Autodesk Fusion 360 part; units mm, degrees
(part 2 of 2)
  constraint perpendicular L106 L211
  constraint horizontal L241
  constraint coincident L210 L241.end
  constraint perpendicular L210 L242
  constraint coincident L210 L243.start
  constraint perpendicular L233 L243
  constraint coincident L233 L243.end
  constraint concentric A1 A243
  constraint concentric A4 A245
  constraint concentric A3 A246
  constraint tangent A134 L244
  constraint tangent L244 A247
  constraint tangent L245 A247
  constraint tangent L113 A248
  constraint tangent L116 A248
  constraint tangent L117 A249
  constraint tangent L120 A249
  constraint tangent L133 A250
  constraint tangent L132 A250
  constraint tangent L178 A251
  constraint tangent L177 A251
  constraint tangent L172 A252
  constraint tangent L171 A252
  constraint tangent L246 A253
  constraint tangent L185 A253
  constraint tangent L247 A254
  constraint tangent L248 A254
  constraint tangent L110 A255
  constraint tangent L242 A255
  constraint tangent L109 A256
  constraint tangent L110 A256
  constraint tangent L108 A257
  constraint tangent L241 A257
  constraint tangent L106 A258
  constraint tangent L107 A258
  measures "d1" diameter of A0
  measures "d2" diameter of A1
  measures "d3" diameter of A2
  measures "d4" diameter of A3
  measures "d5" diameter of A4
  measures "d9" diameter of A111
  measures "d12" diameter of A112
  measures "d255" diameter of A243
  measures "d256" diameter of A244
  measures "d257" diameter of A245
  measures "d259" diameter of A246
extrude "Extrude1" add sketch "mriya" along normal blind 10.6 contours L196 A199 L197 A200 L198 A201 L199 A202 L200 A203 L201 A204 L202 A205 L203 A206 L204 A207 L205 A208 L206 A209 L207 A210 L208 A211 L209 A212 L210 L211 A214 L212 A215 L213 A216 L214 A217 L215 A218 L216 A219 L217 A220 L218 L219 L220 A221 L221 A222 L222 L223 L224 L225 L226 L227 L228 L229 L230 L231 L232 L233 A224 L234 L235 L236 L237 L238 L239 A225 A226 A227 A228 A229 A230 A231 A232 L240 A233 A234 A235 A236 A237 A238 A239 A240 A241 A242 L243 picked at (-141.416666, 51.759867) makes body 1
extrude "Extrude2" add sketch "mriya" along normal blind 17.1 contours L210 A213 L211 L232 A223 L233 L240 L243 picked at (-5.283334, 44.5932) bodies 1
extrude "Extrude3" add sketch "mriya" along normal blind 3.7 contours L106 L107 L108 A113 L109 L110 L196 A199 L197 A200 L198 A201 L199 A202 L200 A203 L201 A204 L202 A205 L203 A206 L204 A207 L205 A208 L206 A209 L207 A210 L208 A211 L209 A212 L210 L211 A214 L212 A215 L213 A216 L214 A217 L215 A218 L216 A219 L217 A220 L241 L242 A255 A256 A257 A258 | L106 L107 L108 A113 L210 A213 L211 L241 A257 A258 | L109 L110 L210 L242 A255 A256 | A115 | A116 | A117 | A118 picked at (-84.826309, 24.168075) picked at (-7.216667, 50.959867) picked at (-7.216666, 8.059867) picked at (-64.728451, 82.79316) picked at (-45.728484, 78.29313) picked at (-25.071567, 2.493271) picked at (-44.071558, 4.793248) bodies 1
extrude "Extrude6" add sketch "mriya" along normal blind 1 from surface at 14.3 contours L106 L107 L108 A113 L210 A213 L211 L241 A257 A258 picked at (-7.216667, 50.959867) bodies 1
extrude "Extrude7" add sketch "mriya" along normal blind 1 from surface at 7.8 contours L109 L110 L210 L242 A255 A256 picked at (-7.216666, 8.059867) bodies 1
sketch "power-switch" plane through (-4.449999, 0, 0) normal (1, 0, 0) x (0, 1, 0)
  line L0 (19.1932, 0) -> (76.4932, 0)
  line L1 (76.4932, 0) -> (76.4932, 16.8)
  line L2 (76.4932, 16.8) -> (19.1932, 16.8)
  line L3 (19.1932, 16.8) -> (19.1932, 10.5)
  line L4 (36.0932, 5.1) -> (25.6932, 5.1)
  line L5 (25.6932, 5.1) -> (25.6932, 8)
  line L6 (25.6932, 8) -> (36.0932, 8)
  line L7 (36.0932, 8) -> (36.0932, 5.1)
  line L8 (37.4932, 3.55) -> (24.2932, 3.55)
  line L9 (23.8932, 3.95) -> (23.8932, 9.15)
  line L10 (24.2932, 9.55) -> (37.4932, 9.55)
  line L11 (37.8932, 9.15) -> (37.8932, 3.95)
  line L12 (19.1932, 10.5) -> (19.1932, 0)
  line L13 (1.9932, 0) -> (76.4932, 0)
  line L14 (76.4932, 0) -> (76.4932, 17.1)
  line L15 (76.4932, 17.1) -> (19.2932, 17.1)
  line L16 (19.2932, 17.1) -> (19.2932, 10.6)
  line L17 (19.2932, 10.6) -> (1.9932, 10.6)
  line L18 (1.9932, 10.6) -> (1.9932, 0)
  arc A0 (24.2932, 9.55) -> (23.8932, 9.15) centre (24.2932, 9.15) ccw
  arc A1 (37.8932, 9.15) -> (37.4932, 9.55) centre (37.4932, 9.15) ccw
  arc A2 (23.8932, 3.95) -> (24.2932, 3.55) centre (24.2932, 3.95) ccw
  arc A3 (37.4932, 3.55) -> (37.8932, 3.95) centre (37.4932, 3.95) ccw
  constraint perpendicular L4 L5
  constraint vertical L5
  constraint perpendicular L5 L6
  constraint vertical L7
  constraint tangent L10 A0
  constraint tangent L9 A0
  constraint tangent L11 A1
  constraint tangent L10 A1
  constraint tangent L9 A2
  constraint tangent L8 A2
  constraint tangent L8 A3
  constraint tangent L11 A3
extrude "Extrude8" cut sketch "power-switch" against normal blind 2.5 contours L4 L5 L6 L7 picked at (32.626533, 6.066667) bodies 1
extrude "Extrude9" cut sketch "power-switch" against normal blind 1 contours L8 L9 L10 L11 A0 A1 A2 A3 picked at (24.4932, 7.033333) bodies 1
chamfer "Chamfer5" distance 0.8 angle 45 4 edges at (-6.949999, 30.8932, 5.1) (-6.949999, 36.0932, 6.55) (-6.949999, 30.8932, 8) (-6.949999, 25.6932, 6.55) on bodies 1
chamfer "Chamfer9" distance 1 angle 45 8 edges at (-4.449999, 37.8932, 6.55) (-4.45, 37.776043, 3.667157) (-4.449999, 30.8932, 3.55) (-4.45, 24.010357, 3.667157) (-4.449999, 23.8932, 6.55) (-4.45, 24.010357, 9.432843) (-4.449999, 30.8932, 9.55) (-4.45, 37.776043, 9.432843) on bodies 1
sketch "usb-c" plane through (0, 80.6432, 0) normal (0, 1, 0) x (-1, 0, 0)
  line L0 (3.6, 0) -> (36.129542, 0)
  line L1 (3.6, 16.7) -> (3.6, 0)
  line L2 (21.20025, 10.9) -> (21.20025, 10.1)
  arc A0 (21.20025, 10.9) -> (19.80025, 12.3) centre (19.80025, 10.9) ccw
  line L3 (11.80025, 10.1) -> (11.80025, 10.9)
  line L4 (19.80025, 8.7) -> (13.20025, 8.7)
  line L5 (21.20025, 7.25) -> (11.80025, 7.25)
  arc A1 (11.80025, 10.1) -> (13.20025, 8.7) centre (13.20025, 10.1) ccw
  line L6 (22.20025, 12.75) -> (22.20025, 8.25)
  line L7 (11.80025, 13.75) -> (21.20025, 13.75)
  arc A2 (13.20025, 12.3) -> (11.80025, 10.9) centre (13.20025, 10.9) ccw
  arc A3 (19.80025, 8.7) -> (21.20025, 10.1) centre (19.80025, 10.1) ccw
  line L8 (10.80025, 8.25) -> (10.80025, 12.75)
  line L9 (13.20025, 12.3) -> (19.80025, 12.3)
  line L10 (8.600001, 0) -> (25.9, 0)
  line L11 (25.9, 10.5) -> (25.9, 16.8)
  line L12 (25.9, 16.8) -> (8.600001, 16.8)
  line L13 (8.600001, 16.8) -> (8.600001, 0)
  line L14 (25.9, 0) -> (25.9, 10.5)
  line L15 (8.600001, 0) -> (41.088119, 0)
  line L16 (41.088119, 0) -> (41.088119, 10.6)
  line L17 (41.088119, 10.6) -> (25.8, 10.6)
  line L18 (25.8, 10.6) -> (25.8, 17.1)
  line L19 (25.8, 17.1) -> (8.600001, 17.1)
  line L20 (8.600001, 17.1) -> (8.600001, 0)
  arc A4 (11.80025, 13.75) -> (10.80025, 12.75) centre (11.80025, 12.75) ccw
  arc A5 (22.20025, 12.75) -> (21.20025, 13.75) centre (21.20025, 12.75) ccw
  arc A6 (10.80025, 8.25) -> (11.80025, 7.25) centre (11.80025, 8.25) ccw
  arc A7 (21.20025, 7.25) -> (22.20025, 8.25) centre (21.20025, 8.25) ccw
  constraint tangent L3 A2
  constraint tangent A2 L9
  constraint tangent A0 L9
  constraint tangent L2 A0
  constraint tangent L4 A3
  constraint tangent L2 A3
  constraint tangent L4 A1
  constraint tangent L3 A1
  constraint perpendicular L6 L7
  constraint perpendicular L5 L8
  constraint horizontal L5
  constraint perpendicular L5 L6
  constraint tangent L7 A4
  constraint tangent L8 A4
  constraint tangent L6 A5
  constraint tangent L7 A5
  constraint tangent L8 A6
  constraint tangent L5 A6
  constraint tangent L5 A7
  constraint tangent L6 A7
extrude "Extrude10" cut sketch "usb-c" against normal blind 2.5 contours L2 A0 L3 L4 A1 A2 A3 L9 picked at (15.40025, 11.1) bodies 1
extrude "Extrude11" cut sketch "usb-c" against normal blind 1 contours L5 L6 L7 L8 A4 A5 A6 A7 picked at (15.40025, 7.733333) bodies 1
chamfer "Chamfer10" distance 1 angle 45 8 edges at (-22.20025, 80.6432, 10.5) (-21.907357, 80.6432, 7.542893) (-16.50025, 80.6432, 7.25) (-11.093143, 80.6432, 7.542893) (-10.80025, 80.6432, 10.5) (-11.093143, 80.6432, 13.457107) (-16.50025, 80.6432, 13.75) (-21.907357, 80.6432, 13.457107) on bodies 1
chamfer "Chamfer4" distance 1 angle 45 90 edges at (-33.44406, 80.6432, 10.6) (-41.470803, 80.71932, 10.6) (-42.359441, 81.500307, 10.6) (-43.896925, 82.71484, 10.6) (-51.46655, 82.943201, 10.6) (-58.272149, 83.019604, 10.6) (-60.260642, 84.900676, 10.6) (-62.896988, 87.214745, 10.6) (-73.400145, 87.443199, 10.6) (-83.903077, 87.214838, 10.6) (-86.040561, 85.400306, 10.6) (-87.529198, 84.019319, 10.6) (-94.833454, 83.943199, 10.6) (-102.903076, 83.714837, 10.6) (-107.217336, 79.723529, 10.6) (-111.044961, 76.05738, 10.6) (-116.187006, 75.9432, 10.6) (-121.903076, 75.714838, 10.6) (-123.440559, 74.500307, 10.6) (-124.329196, 73.71932, 10.6) (-131.40594, 73.6432, 10.6) (-141.034493, 72.427693, 10.6) (-142.25, 42.8932, 10.6) (-141.034493, 13.358707, 10.6) (-120.382982, 12.1432, 10.6) (-100.94415, 12.485634, 10.6) (-96.434572, 16.509865, 10.6) (-92.737435, 19.99135, 10.6) (-84.585569, 20.143201, 10.6) (-75.68512, 19.734247, 10.6) (-70.518243, 11.420229, 10.6) (-65.168056, 2.920317, 10.6) (-56.057903, 2.443204, 10.6) (-48.329196, 2.367084, 10.6) (-47.440558, 1.586096, 10.6) (-45.903073, 0.371562, 10.6) (-37.233452, 0.143202, 10.6) (-29.34028, 0.069542, 10.6) (-28.450122, -0.712016, 10.6) (-26.904053, -1.929959, 10.6) (-17.179837, -2.156801, 10.6) (-5.665506, -0.941293, 10.6) (-4.45, 10.6432, 10.6) (-17.200001, 80.6432, 17.1) (-4.450001, 47.8932, 17.1) (-5.665508, 79.427693, 17.1) (-4.45, 39.2432, 0) (-5.665508, 79.427693, 0) (-24.84406, 80.6432, 0) (-41.470803, 80.71932, 0) (-42.359441, 81.500307, 0) (-43.896925, 82.71484, 0) (-51.46655, 82.943201, 0) (-58.272149, 83.019604, 0) (-60.260642, 84.900676, 0) (-62.896988, 87.214745, 0) (-73.400145, 87.443199, 0) (-83.903077, 87.214838, 0) (-86.040561, 85.400306, 0) (-87.529198, 84.019319, 0) (-94.833454, 83.943199, 0) (-102.903076, 83.714837, 0) (-107.217336, 79.723529, 0) (-111.044961, 76.05738, 0) (-116.187006, 75.9432, 0) (-121.903076, 75.714838, 0) (-123.440559, 74.500307, 0) (-124.329196, 73.71932, 0) (-131.40594, 73.6432, 0) (-141.034493, 72.427693, 0) (-142.25, 42.8932, 0) (-141.034493, 13.358707, 0) (-120.382982, 12.1432, 0) (-100.94415, 12.485634, 0) (-96.434572, 16.509865, 0) (-92.737435, 19.99135, 0) (-84.585569, 20.143201, 0) (-75.68512, 19.734247, 0) (-70.518243, 11.420229, 0) (-65.168056, 2.920317, 0) (-56.057903, 2.443204, 0) (-48.329196, 2.367084, 0) (-47.440558, 1.586096, 0) (-45.903073, 0.371562, 0) (-37.233452, 0.143202, 0) (-29.34028, 0.069542, 0) (-28.450122, -0.712016, 0) (-26.904053, -1.929959, 0) (-17.179837, -2.156801, 0) (-5.665506, -0.941293, 0) on bodies 1
chamfer "Chamfer11" distance 0.79 angle 45 4 edges at (-6.950001, 57.2432, 14.3) (-7.433275, 77.659926, 14.3) (-14.850001, 78.1432, 14.3) (-6.95, 9.5932, 7.8) on bodies 1
fillet "Fillet27" radius 1.2 1 edges at (-4.45, 19.2932, 12.85) on bodies 1
chamfer "Chamfer6" distance 1 angle 45 2 edges at (-6.3, 19.2932, 17.1) (-5.549648, 19.297403, 17.1) on bodies 1
extrude "Extrude12" add sketch "mriya" along normal blind 1.7 contours A2 | L113 L114 L115 L116 A119 A120 A121 A248 | L117 A122 L118 A123 L119 A124 L120 A249 | A125 L121 A126 L122 A127 L123 A128 L124 | A129 L125 A130 L126 A131 L127 A132 L128 | A133 L129 A134 A135 L130 L244 L245 A247 | A136 L131 A137 L132 L133 A138 L134 A250 | A139 L135 A140 L136 A141 L137 A142 L138 | A143 L139 A144 L140 A145 L141 A146 L142 | A147 L143 A148 L144 A149 L145 A150 L146 | A151 L147 A152 L148 A153 L149 A154 L150 | A155 L151 A156 L152 A157 L153 A158 L154 | A159 L155 A160 L156 A161 L157 A162 L158 | A163 L159 A164 L160 A165 L161 A166 L162 | A167 L163 A168 L164 A169 L247 L248 A254 | A170 L165 A171 L166 A172 L167 A173 L168 | A174 L169 A175 L170 A176 L171 L172 A252 | A177 L173 A178 L174 A179 L175 A180 L176 | A181 L177 L178 A182 L179 A183 L180 A251 | A184 L181 A185 L182 A186 L183 A187 L184 | A188 L185 A189 L186 A190 L187 L246 A253 | A191 L188 A192 L189 A193 L190 A194 L191 | A195 L192 A196 L193 A197 L194 A198 L195 picked at (-69.227405, 21.993301) picked at (-128.4, 64.226533) picked at (-128.4, 45.226533) picked at (-128.233333, 26.226533) picked at (-109.233333, 66.526533) picked at (-113.4, 42.859867) picked at (-113.4, 23.859867) picked at (-90.233333, 74.526533) picked at (-94.566667, 55.526533) picked at (-94.566667, 36.526533) picked at (-75.566667, 40.026533) picked at (-71.233333, 59.026533) picked at (-75.566667, 78.026533) picked at (-52.233333, 35.526533) picked at (-52.4, 49.859867) picked at (-52.233333, 73.526533) picked at (-52.4, 11.859867) picked at (-33.233333, 14.226533) picked at (-37.4, 33.226533) picked at (-37.566667, 52.226533) picked at (-37.4, 71.226533) picked at (-18.566667, 11.926533) picked at (-19.233333, 56.559867) bodies 1
sketch "bottom" plane through (0, 0, 0) normal (0, 0, -1) x (1, 0, 0)
  circle A0 centre (-44.9, -22.5432) radius 1.6
  circle A1 centre (-120.9, -34.5432) radius 1.6
  circle A2 centre (-120.9, -53.5432) radius 1.6
  circle A3 centre (-44.9, -60.5432) radius 1.6
  line L0 (-5.450001, -76.4932) -> (-5.449999, -1.9932)
  arc A4 (-5.449999, -1.9932) -> (-8.6, 1.156801) centre (-8.6, -1.9932) ccw
  line L1 (-8.6, 1.156801) -> (-25.759674, 1.156802)
  arc A5 (-25.759674, 1.156802) -> (-27.170137, 0.574756) centre (-25.759674, -0.843198) ccw
  line L2 (-27.170137, 0.574756) -> (-28.319644, -0.568678)
  arc A6 (-29.711881, -1.143202) -> (-28.319644, -0.568678) centre (-29.711881, 0.830953) ccw
  line L3 (-29.711881, -1.143202) -> (-44.755022, -1.143201)
  arc A7 (-44.755022, -1.143201) -> (-46.169236, -1.728987) centre (-44.755022, -3.143201) ccw
  line L4 (-46.169236, -1.728987) -> (-47.297666, -2.857418)
  arc A8 (-48.71188, -3.443204) -> (-47.297666, -2.857418) centre (-48.71188, -1.443204) ccw
  line L5 (-48.71188, -3.443204) -> (-63.403927, -3.443204)
  arc A9 (-63.403927, -3.443204) -> (-65.580565, -4.71347) centre (-63.403927, -5.943204) ccw
  line L6 (-65.580565, -4.71347) -> (-73.71461, -19.110776)
  arc A10 (-77.19723, -21.143201) -> (-73.71461, -19.110776) centre (-77.19723, -17.143201) ccw
  line L7 (-77.19723, -21.143201) -> (-91.973907, -21.143201)
  arc A11 (-94.091778, -20.266106) -> (-91.973907, -21.143201) centre (-91.973907, -18.147703) ccw
  line L8 (-94.091778, -20.266106) -> (-100.191401, -14.168016)
  arc A12 (-100.191401, -14.168016) -> (-102.665964, -13.1432) centre (-102.665964, -16.6432) ccw
  line L9 (-102.665964, -13.1432) -> (-138.1, -13.143201)
  arc A13 (-138.1, -13.143201) -> (-141.25, -16.2932) centre (-138.1, -16.2932) ccw
  line L10 (-141.25, -16.2932) -> (-141.25, -69.4932)
  arc A14 (-141.25, -69.4932) -> (-138.1, -72.6432) centre (-138.1, -69.4932) ccw
  line L11 (-138.1, -72.6432) -> (-124.711879, -72.6432)
  arc A15 (-123.297666, -73.228986) -> (-124.711879, -72.6432) centre (-124.711879, -74.6432) ccw
  line L12 (-123.297666, -73.228986) -> (-122.169239, -74.357413)
  arc A16 (-122.169239, -74.357413) -> (-120.755025, -74.9432) centre (-120.755025, -72.9432) ccw
  line L13 (-120.755025, -74.9432) -> (-111.618986, -74.9432)
  arc A17 (-109.851219, -75.675433) -> (-111.618986, -74.9432) centre (-111.618986, -77.4432) ccw
  line L14 (-109.851219, -75.675433) -> (-103.169239, -82.357412)
  arc A18 (-103.169239, -82.357412) -> (-101.755026, -82.943199) centre (-101.755026, -80.943199) ccw
  line L15 (-101.755026, -82.943199) -> (-87.911882, -82.943199)
  arc A19 (-86.497668, -83.528985) -> (-87.911882, -82.943199) centre (-87.911882, -84.943199) ccw
  line L16 (-86.497668, -83.528985) -> (-84.169241, -85.857413)
  arc A20 (-84.169241, -85.857413) -> (-82.755027, -86.443199) centre (-82.755027, -84.443199) ccw
  line L17 (-82.755027, -86.443199) -> (-64.045264, -86.4432)
  arc A21 (-64.045264, -86.4432) -> (-62.63082, -85.857183) centre (-64.045264, -84.4432) ccw
  line L18 (-62.63082, -85.857183) -> (-59.304908, -82.530187)
  arc A22 (-57.888124, -81.943201) -> (-59.304908, -82.530187) centre (-57.888124, -83.946509) ccw
  line L19 (-57.888124, -81.943201) -> (-45.044975, -81.943201)
  arc A23 (-45.044975, -81.943201) -> (-43.630762, -81.357414) centre (-45.044975, -79.943201) ccw
  line L20 (-43.630762, -81.357414) -> (-42.502333, -80.228986)
  arc A24 (-41.088119, -79.643199) -> (-42.502333, -80.228986) centre (-41.088119, -81.643199) ccw
  line L21 (-41.088119, -79.643199) -> (-8.600001, -79.6432)
  arc A25 (-8.600001, -79.6432) -> (-5.450001, -76.4932) centre (-8.600001, -76.4932) ccw
  circle A26 centre (-44.9, -60.5432) radius 2
  circle A27 centre (-44.9, -22.5432) radius 2
  circle A28 centre (-120.9, -53.5432) radius 2
  circle A29 centre (-120.9, -34.5432) radius 2
  circle A30 centre (-10.950001, -74.1432) radius 4
  circle A31 centre (-10.949999, -4.343199) radius 4
  circle A32 centre (-61.653156, -8.943204) radius 4
  circle A33 centre (-73.400145, -80.943199) radius 4
  circle A34 centre (-135.75, -67.1432) radius 4
  circle A35 centre (-135.75, -18.643201) radius 4
  dimension "d261" = 4
  dimension "d262" = 4
  dimension "d263" = 4
  dimension "d264" = 4
  dimension "d265" = 8
  dimension "d266" = 8
  dimension "d267" = 8
  dimension "d268" = 8
  dimension "d269" = 8
  dimension "d270" = 8
  dimension "d271" = 5.5
  dimension "d272" = 5.5
  dimension "d273" = 5.5
  dimension "d274" = 5.5
  dimension "d275" = 5.5
  dimension "d276" = 5.5
  dimension "d277" = 5.5
  dimension "d278" = 5.5
  dimension "d279" = 5.5
  dimension "d280" = 5.5
  dimension "d281" = 5.5
  constraint concentric A3 A26
  constraint concentric A0 A27
  constraint concentric A2 A28
  constraint concentric A1 A29
  measures "d261" diameter of A26
  measures "d262" diameter of A27
  measures "d263" diameter of A28
  measures "d264" diameter of A29
  measures "d265" diameter of A30
  measures "d266" diameter of A31
  measures "d267" diameter of A32
  measures "d268" diameter of A33
  measures "d269" diameter of A34
  measures "d270" diameter of A35
  measures "d279" distance of L10 A34.centre
  measures "d280" distance of L11 A34.centre
extrude "Extrude13" add sketch "mriya" along normal blind 1.7 contours A0 | A1 | A3 | A4 picked at (-120.872599, 54.972525) picked at (-120.872599, 33.113875) picked at (-43.472624, 22.463711) picked at (-46.000407, 59.630607) bodies 1
extrude "Extrude14" cut sketch "bottom" against normal blind 0.8 contours A0 | A1 | A2 | A3 | A26 | A27 | A28 | A29 | A30 | A31 | A32 | A33 | A34 | A35 picked at (-44.633333, -21.766914) picked at (-121.166667, -35.46789) picked at (-120.633333, -54.46789) picked at (-44.633333, -59.766914) picked at (-46.380188, -59.413767) picked at (-43.604678, -23.880628) picked at (-119.604678, -52.205772) picked at (-122.380188, -35.672633) picked at (-10.850361, -75.295925) picked at (-9.972597, -3.436302) picked at (-62.012246, -8.943204) picked at (-75.385253, -81.58045) picked at (-137.855417, -68.307559) picked at (-137.320791, -19.550098) bodies 1
mirror "Mirror1" about plane through (0, 0, 0) normal (1, 0, 0) of bodies 1 makes body 2
named bodies: "Left", "Right"
